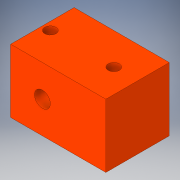
# Autodesk Inventor part: ElevDriveBlock
Saved by Autodesk Inventor 2019 (Build 230136000, 136)
## iProperties
Created: 2019-10-06
Part Number: ElevDriveBlock
Material: Generic
Document SubType Name: Modeling
Designer: james
Density: 1 g/cm^3
Appearance: Default(1)
Author: james
Autodesk Inventor part; units mm, degrees
ref_plane "YZ Plane" through (0, 0, 0) normal (1, 0, 0) x (0, 1, 0)
ref_plane "XZ Plane" through (0, 0, 0) normal (0, 1, 0) x (-1, 0, 0)
ref_plane "XY Plane" through (0, 0, 0) normal (0, 0, 1) x (1, 0, 0)
sketch "Sketch1" plane through (0, 0, 0) normal (0, 1, 0) x (-1, 0, 0)
  line L0 (26.3596, 46.3409) -> (-11.7404, 46.3409)
  line L1 (-11.7404, 46.3409) -> (-11.7404, 20.9409)
  line L2 (-11.7404, 20.9409) -> (26.3596, 20.9409)
  line L3 (26.3596, 20.9409) -> (26.3596, 46.3409)
  point P0 (0, 0)
  dimension "d0" = 25.4
  dimension "d1" = 38.1
  constraints: 8 end point, 2 parallel, 1 horizontal, 1 perpendicular
  measures "d0" distance of L2.end L0.start
  measures "d1" distance of L1.end L2.end
extrude "Extrusion1" add sketch "Sketch1" along normal blind 25.4
sketch "Sketch2" plane through (0, 25.4, 0) normal (0, 1, 0) x (1, 0, 0)
  line L0 (-26.3596, -46.3409) -> (11.7404, -46.3409) projected
  line L1 (-26.3596, -20.9409) -> (-26.3596, -46.3409) projected
  point P0 (0, 0)
  point P1 (-23.1846, -33.6409)
  point P2 (2.2154, -33.6409)
  dimension "d4" = 0
  dimension "d5" = 12.7
  dimension "d6" = 3.175
  dimension "d7" = 25.4
  measures "d4" vertical distance of point (2.215, -33.641) point (-23.185, -33.641)
  measures "d5" distance from line of L0 point (-23.185, -33.641)
  measures "d6" distance from line of L1 point (-23.185, -33.641)
  measures "d7" distance of point (-23.185, -33.641) point (2.215, -33.641)
hole "Hole1" at (-23.1846, 25.4, 33.6409) at (2.2154, 25.4, 33.6409) direction (0, -1, 0) diameter 4.4958 end through all clearance for "Flat Head Machine Screw (82)" size "#8" standard "Ansi Unified Screw Threads"
sketch "Sketch3" plane through (-26.3596, 0, 46.3409) normal (0, 0, 1) x (1, 0, 0)
  line L0 (0, 0) -> (0, 25.4) projected
  line L1 (0, 25.4) -> (38.1, 25.4) projected
  point P0 (26.3596, 0)
  point P1 (12.7, 12.7)
  dimension "d15" = 12.7
  dimension "d16" = 12.7
  measures "d15" distance from line of L0 point (12.7, 12.7)
  measures "d16" distance from line of L1 point (12.7, 12.7)
hole "Hole2" at (-13.6596, 12.7, 46.3409) direction (0, 0, -1) diameter 6.35 end through all
body "Solid1"
